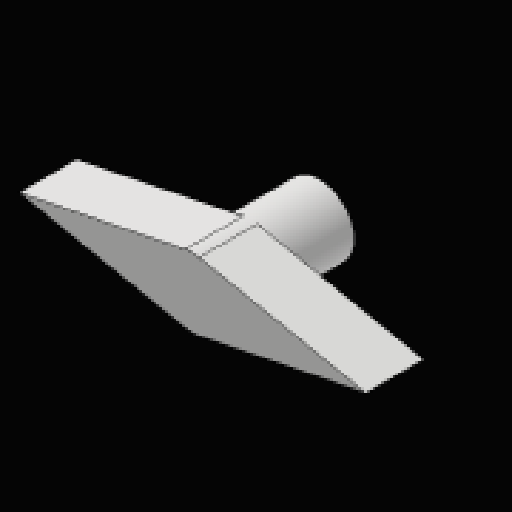
# Autodesk Inventor part: Leg
Saved by Autodesk Inventor 2023.2 (Build 272271030, 271C)
## iProperties
Created: 2023-11-11
Part Number: Leg
Material: Generic
Document SubType Name: Modeling
Designer: robpl
Density: 1 g/cm^3
Appearance: Default
Author: robpl
Autodesk Inventor part; units mm, degrees
ref_plane "YZ Plane" through (0, 0, 0) normal (1, 0, 0) x (0, 1, 0)
ref_plane "XZ Plane" through (0, 0, 0) normal (0, 1, 0) x (-1, 0, 0)
ref_plane "XY Plane" through (0, 0, 0) normal (0, 0, 1) x (1, 0, 0)
sketch "Sketch1" plane through (0, 0, 0) normal (0, 0, 1) x (1, 0, 0)
  circle A0 centre (0, 0) radius 3.5
  dimension "d0" = 7
  constraints: 1 centre point, 1 coincident
  measures "d0" diameter of A0
extrude "Extrusion1" add sketch "Sketch1" along normal blind 9
sketch "Sketch2" plane through (0, 0, 9) normal (0, 0, 1) x (1, 0, 0)
  circle A0 centre (0, 0) radius 3.5 projected
  circle A1 centre (0, 0) radius 3.5 projected
  line L0 (-0.8167, 3.4034) -> (-15, 0)
  line L1 (-15, 0) -> (-0.8167, -3.4034)
  line L2 (0.8167, 3.4034) -> (15, 0)
  line L3 (15, 0) -> (0.8167, -3.4034)
  circle A2 centre (0, 0) radius 3.5 projected
  circle A3 centre (0, 0) radius 3.5
  point P0 (0.8167, 3.4034)
  point P1 (-0.8167, 3.4034)
  point P2 (-0.8167, -3.4034)
  point P3 (0.8167, -3.4034)
  dimension "d3" = 30
  constraints: 8 end point, 4 point on circle, 4 tangent, 2 parallel, 1 coincident, 1 horizontal alignment, 3 other
  measures "d3" distance of L0.end L2.end
extrude "Extrusion2" add sketch "Sketch2" along normal blind 5
body "Solid1"
